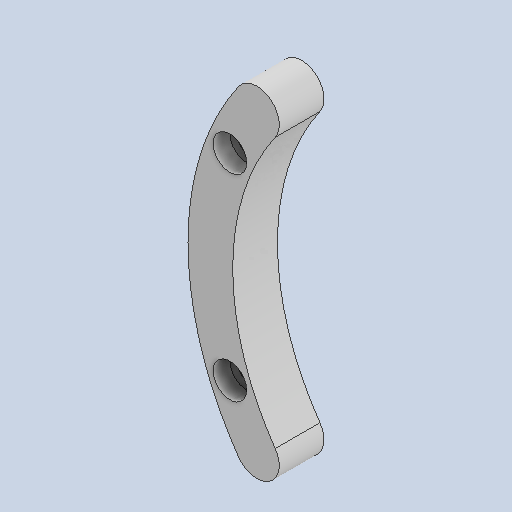
# Autodesk Inventor part: legparts_10
Saved by Autodesk Inventor 2024.3 (Build 283343000, 343)
## iProperties
Created: 2025-01-05
Part Number: legparts_10
Material: 一般
Document SubType Name: Modeling
Designer: 佐藤智貴
Density: 1 g/cm^3
Appearance: 既定
Author: 佐藤智貴
Autodesk Inventor part; units mm, degrees
ref_plane "YZ Plane" through (0, 0, 0) normal (1, 0, 0) x (0, 1, 0)
ref_plane "XZ Plane" through (0, 0, 0) normal (0, 1, 0) x (-1, 0, 0)
ref_plane "XY Plane" through (0, 0, 0) normal (0, 0, 1) x (1, 0, 0)
sketch "スケッチ1" plane through (0, 0, 0) normal (0, 0, 1) x (1, 0, 0)
  circle A0 centre (0, 0) radius 46
  circle A1 centre (0, 0) radius 50
  circle A2 centre (0, 0) radius 42
  line L0 (0, 0) -> (0, 54.8528)
  line L1 (0, 0) -> (-20.7697, 50.1426)
  circle A3 centre (-17.6034, 42.4985) radius 1.5
  circle A4 centre (-42.4985, 17.6034) radius 1.5
  circle A5 centre (-42.4985, -17.6034) radius 1.5
  circle A6 centre (-17.6034, -42.4985) radius 1.5
  circle A7 centre (17.6034, -42.4985) radius 1.5
  circle A8 centre (42.4985, -17.6034) radius 1.5
  circle A9 centre (42.4985, 17.6034) radius 1.5
  circle A10 centre (17.6034, 42.4985) radius 1.5
  line L2 (0, 0) -> (-55.1659, -46.2897)
  line L3 (-55.1659, -46.2897) -> (-55.1659, 46.2897)
  line L4 (-55.1659, 46.2897) -> (0, 0)
  line L5 (0, 0) -> (-76.7662, 0)
  point P0 (-32.1739, -26.9971)
  point P1 (-32.1739, 26.9971)
  point P2 (-38.3022, 32.1394)
  point P3 (-38.3022, -32.1394)
  dimension "d0" = 92
  dimension "d1" = 100
  dimension "d2" = 84
  dimension "d3" = 22.5
  dimension "d4" = 3
  dimension "d7" = 360
  dimension "d9" = 80
  dimension "d10" = 40
  constraints: 12 end point, 10 centre point, 2 coincident, 2 vertical, 1 horizontal, 1 point on line, 20 other
  measures "d1" diameter of A1
  measures "d2" diameter of A2
  measures "d3" angle of L0 L1
  measures "d4" diameter of A3
  measures "d9" angle of L4 L2
  measures "d10" angle of L2 L5
extrude "押し出し1" add sketch "スケッチ1" along normal blind 8 contours L2 A1 L5 A0 A5 | A0 A5 L5 A2 L2 | A2 L5 A0 A4 L4 | L4 A0 A4 L5 A1
fillet "フィレット1" radius 4 4 edges at (-32.1739, -26.9971, 4) (-38.3022, -32.1394, 4) (-38.3022, 32.1394, 4) (-32.1739, 26.9971, 4)
sketch "スケッチ2" plane through (0, 0, 8) normal (0, 0, 1) x (1, 0, 0)
  circle A0 centre (-42.4985, -17.6034) radius 1.5 projected
  circle A1 centre (-42.4985, -17.6034) radius 3
  circle A2 centre (-42.4985, 17.6034) radius 1.5 projected
  circle A3 centre (-42.4985, 17.6034) radius 3
  point P0 (0, 0)
  dimension "d14" = 6
  dimension "d15" = 6
  constraints: 2 centre point, 2 coincident
  measures "d14" diameter of A3
  measures "d15" diameter of A1
extrude "押し出し2" cut sketch "スケッチ2" against normal blind 3 contours A0 | A1 | A2 | A3
equation "\"d10\" = 0.5 * d9"
